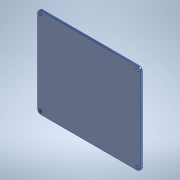
# Autodesk Inventor part: 视空盖1
Saved by Autodesk Inventor 2020 (Build 240168000, 168)
## iProperties
Created: 2021-06-16
Part Number: 视空盖1
Material: 常规
Document SubType Name: Modeling
Designer: dell
Density: 1 g/cm^3
Appearance: 薄片缎光 - 蓝色
Author: dell
Autodesk Inventor part; units mm, degrees
ref_plane "YZ Plane" through (0, 0, 0) normal (1, 0, 0) x (0, 1, 0)
ref_plane "XZ Plane" through (0, 0, 0) normal (0, 1, 0) x (-1, 0, 0)
ref_plane "工作平面1" through (0, 0, 0) normal (0, 0, 1) x (1, 0, 0)
sketch "草图1" plane through (0, 0, 0) normal (0, 0, 1) x (1, 0, 0)
  circle A0 centre (-97, -84) radius 2.4585 projected
  circle A1 centre (97, 84) radius 2.4585 projected
  circle A2 centre (97, -84) radius 2.4585 projected
  circle A3 centre (-97, 84) radius 2.4585 projected
  line L0 (85, -75) -> (-85, -75) construction
  line L1 (-85, -75) -> (-85, 75) construction
  line L2 (-85, 75) -> (85, 75) construction
  line L3 (85, 75) -> (85, -75) construction
  arc A4 (97, -90) -> (103, -84) centre (97, -84) ccw projected
  line L4 (103, -84) -> (103, 84) projected
  arc A5 (103, 84) -> (97, 90) centre (97, 84) ccw projected
  line L5 (97, 90) -> (-97, 90) projected
  arc A6 (-97, 90) -> (-103, 84) centre (-97, 84) ccw projected
  line L6 (-103, 84) -> (-103, -84) projected
  arc A7 (-103, -84) -> (-97, -90) centre (-97, -84) ccw projected
  line L7 (-97, -90) -> (97, -90) projected
  point P0 (0, 0)
extrude "拉伸1" add sketch "草图1" along normal blind 4
sketch "草图2" plane through (0, 0, 4) normal (0, 0, 1) x (1, 0, 0)
  arc A0 (103, 84) -> (97, 90) centre (97, 84) ccw construction
  line L0 (97, 90) -> (-97, 90) construction
  arc A1 (-97, 90) -> (-103, 84) centre (-97, 84) ccw construction
  line L1 (-103, 84) -> (-103, -84) construction
  arc A2 (-103, -84) -> (-97, -90) centre (-97, -84) ccw construction
  line L2 (-97, -90) -> (97, -90) construction
  arc A3 (97, -90) -> (103, -84) centre (97, -84) ccw construction
  line L3 (103, -84) -> (103, 84) construction
  circle A4 centre (-97, -84) radius 2.4585 construction
  circle A5 centre (97, -84) radius 2.4585 construction
  circle A6 centre (-97, 84) radius 2.4585 construction
  circle A7 centre (97, 84) radius 2.4585 construction
  circle A8 centre (97, 84) radius 2.9585
  circle A9 centre (-97, 84) radius 2.9585
  circle A10 centre (-97, -84) radius 2.9585
  circle A11 centre (97, -84) radius 2.9585
  point P0 (0, 0)
  dimension "d2" = 0.5
  dimension "d3" = 0.5
  dimension "d4" = 0.5
  dimension "d5" = 0.5
  constraints: 4 centre point
  measures "d2" radial gap between concentric circles of A7 A8
  measures "d3" radial gap between concentric circles of A6 A9
  measures "d4" radial gap between concentric circles of A4 A10
  measures "d5" radial gap between concentric circles of A5 A11
extrude "拉伸2" cut sketch "草图2" against normal up to surface (4 mm away)
